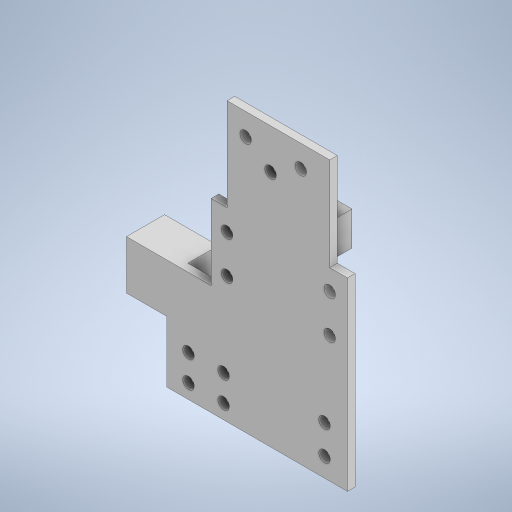
# Autodesk Inventor part: diods low holder
Saved by Autodesk Inventor 2023.1 (Build 271208000, 208)
## iProperties
Created: 2023-04-12
Part Number: diods low holder
Material: Типовые
Document SubType Name: Modeling
Designer: User
Density: 1 g/cm^3
Appearance: По умолчанию
Author: User
Autodesk Inventor part; units mm, degrees
(part 1 of 4)
ref_plane "YZ Plane" through (0, 0, 0) normal (1, 0, 0) x (0, 1, 0)
ref_plane "XZ Plane" through (0, 0, 0) normal (0, 1, 0) x (-1, 0, 0)
ref_plane "XY Plane" through (0, 0, 0) normal (0, 0, 1) x (1, 0, 0)
sketch "Эскиз1" plane through (0, 0, 0) normal (0, 0, 1) x (1, 0, 0)
  arc A0 (16.2316, 29.0119) -> (15.6959, 29.5476) centre (15.6959, 29.0119) ccw
  line L0 (15.6959, 29.5476) -> (-3.717, 29.5476)
  line L1 (-3.717, 29.5476) -> (-3.717, 30.0833)
  line L2 (-3.717, 30.0833) -> (15.6959, 30.0833)
  arc A1 (16.7673, 29.0119) -> (15.6959, 30.0833) centre (15.6959, 29.0119) ccw
  line L3 (-15.01, 19.0821) -> (-15.01, 61.0407)
  arc A2 (-14.6801, 30.0833) -> (-15.7515, 29.0119) centre (-14.6801, 29.0119) ccw
  line L4 (-14.6801, 30.0833) -> (-13.7863, 30.0833)
  line L5 (-13.7863, 30.0833) -> (-13.7863, 29.5488)
  line L6 (-13.7863, 29.5488) -> (-14.6801, 29.5488)
  arc A3 (-14.6801, 29.5488) -> (-15.217, 29.0119) centre (-14.6801, 29.0119) ccw
  arc A4 (-13.6086, 46.5113) -> (-12.5371, 45.4398) centre (-12.5371, 46.5113) ccw
  line L7 (-13.6086, 46.5113) -> (-13.6086, 48.3204)
  arc A5 (-12.5371, 49.3918) -> (-13.6086, 48.3204) centre (-12.5371, 48.3204) ccw
  line L8 (-12.5371, 49.3918) -> (13.531, 49.3918)
  arc A6 (14.6024, 48.3204) -> (13.531, 49.3918) centre (13.531, 48.3204) ccw
  line L9 (14.6024, 48.3204) -> (14.6024, 46.5113)
  arc A7 (13.531, 45.4398) -> (14.6024, 46.5113) centre (13.531, 46.5113) ccw
  line L10 (13.531, 45.4398) -> (-12.5371, 45.4398)
  arc A8 (-13.6083, 35.1179) -> (-12.5369, 34.0465) centre (-12.5369, 35.1179) ccw
  line L11 (-13.6083, 35.1179) -> (-13.6083, 43.4963)
  arc A9 (-12.5369, 44.5677) -> (-13.6083, 43.4963) centre (-12.5369, 43.4963) ccw
  line L12 (-12.5369, 44.5677) -> (13.5311, 44.5677)
  arc A10 (14.6025, 43.4963) -> (13.5311, 44.5677) centre (13.5311, 43.4963) ccw
  line L13 (14.6025, 43.4963) -> (14.6025, 35.1179)
  arc A11 (13.5311, 34.0465) -> (14.6025, 35.1179) centre (13.5311, 35.1179) ccw
  line L14 (13.5311, 34.0465) -> (-12.5369, 34.0465)
  line L15 (12.4115, -40.9097) -> (12.4115, -39.4422)
  line L16 (12.4115, -39.4422) -> (12.1037, -39.4422)
  line L17 (12.1037, -39.4422) -> (11.6041, -40.9521)
  line L18 (4.6702, -39.4422) -> (4.1371, -39.4422)
  line L19 (4.1371, -39.4422) -> (4.1371, -40.9097)
  line L20 (3.0666, -40.5083) -> (3.0666, -39.4422)
  line L21 (3.0666, -39.4422) -> (2.5335, -39.4422)
  line L22 (-3.0712, -39.3084) -> (-3.0712, -39.9752)
  line L23 (-3.0712, -39.9752) -> (-2.2727, -39.9752)
  line L24 (-2.2727, -39.9752) -> (-2.2727, -39.3084)
  line L25 (-2.2727, -40.9097) -> (-2.2727, -40.2429)
  line L26 (-2.2727, -40.2429) -> (-3.0712, -40.2429)
  line L27 (-3.0712, -40.2429) -> (-3.0712, -40.9097)
  line L28 (-8.7049, -39.3084) -> (-8.7049, -40.0957)
  line L29 (-8.7049, -40.0957) -> (-7.8573, -39.2058)
  line L30 (-7.6812, -39.4087) -> (-8.2187, -39.973)
  line L31 (-8.2187, -39.973) -> (-7.6678, -40.8227)
  line L32 (-9.7486, -40.5083) -> (-9.7486, -39.4422)
  line L33 (-9.7486, -39.4422) -> (-10.2817, -39.4422)
  line L34 (-6.4778, -35.8752) -> (-6.9921, -35.1051)
  line L35 (-6.9921, -35.1051) -> (-7.5063, -35.8752)
  line L36 (-7.7811, -35.6929) -> (-7.1907, -34.8085)
  line L37 (-7.1907, -34.8085) -> (-7.7811, -33.9242)
  line L38 (-7.5063, -33.7419) -> (-6.9921, -34.512)
  line L39 (-6.9921, -34.512) -> (-6.4778, -33.7419)
  line L40 (-6.203, -33.9242) -> (-6.7934, -34.8085)
  line L41 (-6.7934, -34.8085) -> (-6.203, -35.6929)
  line L42 (-13.0904, -31.8235) -> (-12.0092, -35.0208)
  line L43 (-12.0092, -35.0208) -> (-10.9279, -31.8235)
  line L44 (9.2465, -26.7019) -> (9.7795, -26.7019)
  line L45 (9.7795, -26.7019) -> (9.7795, -26.1689)
  line L46 (9.7795, -26.1689) -> (9.2465, -26.1689)
  line L47 (9.7795, -27.6364) -> (9.7795, -26.9696)
  line L48 (9.7795, -26.9696) -> (9.4517, -26.9696)
  line L49 (9.4517, -26.9696) -> (8.9588, -27.71)
  line L50 (7.9106, -27.235) -> (7.9106, -26.1689)
  line L51 (7.9106, -26.1689) -> (7.3775, -26.1689)
  line L52 (-0.6337, -27.6364) -> (-0.6337, -26.1689)
  line L53 (-0.6337, -26.1689) -> (-0.9414, -26.1689)
  line L54 (-0.9414, -26.1689) -> (-1.441, -27.6788)
  line L55 (-8.375, -26.1689) -> (-8.908, -26.1689)
  line L56 (-8.908, -26.1689) -> (-8.908, -27.6364)
  line L57 (-9.9785, -27.235) -> (-9.9785, -26.1689)
  line L58 (-9.9785, -26.1689) -> (-10.5116, -26.1689)
  line L59 (7.9308, 57.2595) -> (9.7846, 57.2595)
  line L60 (9.7846, 57.2595) -> (9.7846, 54.4455)
  line L61 (9.7846, 54.4455) -> (9.3105, 54.4455)
  line L62 (9.3105, 54.4455) -> (9.3105, 56.8614)
  line L63 (9.3105, 56.8614) -> (8.3441, 56.8614)
  line L64 (7.3018, 54.4455) -> (7.3018, 54.8588)
  line L65 (7.3018, 54.8588) -> (7.3261, 54.8588)
  line L66 (2.4335, 54.5883) -> (2.4335, 53.4093)
  line L67 (2.4335, 53.4093) -> (1.9594, 53.4093)
  line L68 (1.9594, 53.4093) -> (1.9594, 57.2595)
  line L69 (1.9594, 57.2595) -> (2.4335, 57.2595)
  line L70 (2.4335, 57.2595) -> (2.4335, 56.9648)
  line L71 (-1.6052, 54.4455) -> (-1.6052, 55.7127)
  line L72 (-1.6052, 55.7127) -> (-2.8755, 55.7127)
  line L73 (-2.8755, 55.7127) -> (-2.8755, 54.4455)
  line L74 (-2.8755, 54.4455) -> (-3.3496, 54.4455)
  line L75 (-3.3496, 54.4455) -> (-3.3496, 57.2595)
  line L76 (-3.3496, 57.2595) -> (-2.8755, 57.2595)
  line L77 (-2.8755, 57.2595) -> (-2.8755, 56.1199)
  line L78 (-2.8755, 56.1199) -> (-1.6052, 56.1199)
  line L79 (-1.6052, 56.1199) -> (-1.6052, 57.2595)
  line L80 (-1.6052, 57.2595) -> (-1.1312, 57.2595)
  line L81 (-1.1312, 57.2595) -> (-1.1312, 54.4455)
  line L82 (-1.1312, 54.4455) -> (-1.6052, 54.4455)
  line L83 (-1.0482, 51.8431) -> (-1.3158, 51.8431)
  line L84 (-1.3158, 51.8431) -> (-1.3158, 51.3101)
  line L85 (-1.3158, 51.3101) -> (-1.0482, 51.3101)
  line L86 (-1.3158, 52.7776) -> (-1.3158, 52.1107)
  line L87 (-1.3158, 52.1107) -> (-1.0482, 52.1107)
  line L88 (-7.1926, 51.1763) -> (-7.1926, 52.6438)
  line L89 (-7.1926, 52.6438) -> (-7.7257, 52.6438)
  line L90 (-7.7257, 52.6438) -> (-7.7257, 51.1763)
  line L91 (-6.6574, 52.6438) -> (-6.925, 52.6438)
  line L92 (-6.925, 52.6438) -> (-6.925, 51.1763)
  line L93 (-10.9306, 51.3101) -> (-10.3975, 51.3101)
  line L94 (-10.3975, 51.3101) -> (-10.3975, 52.7776)
  arc A12 (-14.7321, -26.6456) -> (-15.8036, -27.717) centre (-14.7321, -27.717) ccw
  line L95 (-14.7321, -26.6456) -> (-13.7859, -26.6456)
  line L96 (-13.7859, -26.6456) -> (-13.7859, -27.1813)
  line L97 (-13.7859, -27.1813) -> (-14.7321, -27.1813)
  arc A13 (-14.7321, -27.1813) -> (-15.2679, -27.717) centre (-14.7321, -27.717) ccw
  line L98 (-15.2679, -27.717) -> (-15.2679, -55.0248)
  arc A14 (-15.2679, -55.0248) -> (-14.7321, -55.5605) centre (-14.7321, -55.0248) ccw
  line L99 (-14.7321, -55.5605) -> (15.5357, -55.5605)
  arc A15 (15.5357, -55.5605) -> (16.0714, -55.0248) centre (15.5357, -55.0248) ccw
  line L100 (16.0714, -55.0248) -> (16.0714, -27.717)
  arc A16 (16.0714, -27.717) -> (15.5357, -27.1813) centre (15.5357, -27.717) ccw
  line L101 (15.5357, -27.1813) -> (11.1025, -27.1813)
  line L102 (11.1025, -27.1813) -> (11.1025, -26.6456)
  line L103 (11.1025, -26.6456) -> (15.5357, -26.6456)
  arc A17 (16.6071, -27.717) -> (15.5357, -26.6456) centre (15.5357, -27.717) ccw
  line L104 (16.6071, -27.717) -> (16.6071, -55.0248)
  arc A18 (15.5357, -56.0962) -> (16.6071, -55.0248) centre (15.5357, -55.0248) ccw
  line L105 (15.5357, -56.0962) -> (-14.7321, -56.0962)
  arc A19 (-15.8036, -55.0248) -> (-14.7321, -56.0962) centre (-14.7321, -55.0248) ccw
  line L106 (-15.8036, -55.0248) -> (-15.8036, -27.717)
  line L107 (-5.3214, 52.3784) -> (-5.3214, 52.1107)
  line L108 (-5.3214, 52.1107) -> (-4.523, 52.1107)
  line L109 (-4.523, 52.1107) -> (-4.523, 52.3784)
  line L110 (-4.3892, 51.8431) -> (-5.3214, 51.8431)
  line L111 (-5.3214, 51.8431) -> (-5.3214, 51.5777)
  line L112 (-2.3864, 51.1763) -> (-2.3864, 52.3628)
  line L113 (-2.3864, 52.3628) -> (-2.8101, 51.7673)
  line L114 (-3.0287, 51.7673) -> (-3.4524, 52.3628)
  line L115 (-3.4524, 52.3628) -> (-3.4524, 51.1763)
  line L116 (-3.477, 52.8557) -> (-2.9194, 52.0728)
  line L117 (-2.9194, 52.0728) -> (-2.3618, 52.8557)
  line L118 (-7.5979, 55.9407) -> (-6.4553, 54.4455)
  line L119 (-6.4553, 54.4455) -> (-7.0449, 54.4455)
  line L120 (-7.0449, 54.4455) -> (-8.0082, 55.7431)
  line L121 (-8.0082, 55.7431) -> (-8.2422, 55.7431)
  line L122 (-8.2422, 55.7431) -> (-8.2422, 54.4455)
  line L123 (-8.2422, 54.4455) -> (-8.7162, 54.4455)
  line L124 (-8.7162, 54.4455) -> (-8.7162, 57.2595)
  line L125 (-8.7162, 57.2595) -> (-8.2422, 57.2595)
  line L126 (-8.2422, 57.2595) -> (-8.2422, 56.0349)
  line L127 (-6.7774, 57.2595) -> (-6.6498, 57.2595)
  line L128 (-6.6498, 57.2595) -> (-6.6498, 56.8523)
  line L129 (-6.6498, 56.8523) -> (-6.7592, 56.8523)
  line L130 (0.6496, 56.8462) -> (0.6496, 54.4455)
  line L131 (0.6496, 54.4455) -> (0.1756, 54.4455)
  line L132 (0.1756, 54.4455) -> (0.1756, 56.8462)
  line L133 (0.1756, 56.8462) -> (-0.7817, 56.8462)
  line L134 (-0.7817, 56.8462) -> (-0.7817, 57.2595)
  line L135 (-0.7817, 57.2595) -> (1.6069, 57.2595)
  line L136 (1.6069, 57.2595) -> (1.6069, 56.8462)
  line L137 (1.6069, 56.8462) -> (0.6496, 56.8462)
  line L138 (11.2979, 55.7796) -> (10.9454, 55.7796)
  line L139 (10.9454, 55.7796) -> (10.9454, 54.8223)
  line L140 (10.9454, 54.8223) -> (11.2858, 54.8223)
  line L141 (11.456, 54.4455) -> (10.4714, 54.4455)
  line L142 (10.4714, 54.4455) -> (10.4714, 57.2595)
  line L143 (10.4714, 57.2595) -> (10.9454, 57.2595)
  line L144 (10.9454, 57.2595) -> (10.9454, 56.1625)
  line L145 (10.9454, 56.1625) -> (11.4681, 56.1625)
  line L146 (-12.646, -26.0351) -> (-12.646, -26.7019)
  line L147 (-12.646, -26.7019) -> (-11.8475, -26.7019)
  line L148 (-11.8475, -26.7019) -> (-11.8475, -26.0351)
  line L149 (-11.8475, -27.6364) -> (-11.8475, -26.9696)
  line L150 (-11.8475, -26.9696) -> (-12.646, -26.9696)
  line L151 (-12.646, -26.9696) -> (-12.646, -27.6364)
  line L152 (-6.506, -26.1689) -> (-7.039, -26.1689)
  line L153 (-7.039, -26.1689) -> (-7.039, -27.5026)
  line L154 (-7.039, -27.5026) -> (-6.506, -27.5026)
  line L155 (-6.506, -27.7703) -> (-7.039, -27.7703)
  line L156 (-7.039, -27.7703) -> (-7.039, -28.4371)
  line L157 (-4.3716, -27.235) -> (-4.3716, -26.1689)
  line L158 (-4.3716, -26.1689) -> (-4.9046, -26.1689)
  line L159 (0.7023, -26.7019) -> (1.2353, -26.7019)
  line L160 (1.2353, -26.7019) -> (1.2353, -26.1689)
  line L161 (1.2353, -26.1689) -> (0.7023, -26.1689)
  line L162 (1.2353, -27.6364) -> (1.2353, -26.9696)
  line L163 (1.2353, -26.9696) -> (0.9075, -26.9696)
  line L164 (0.9075, -26.9696) -> (0.4146, -27.71)
  line L165 (2.3059, -26.0351) -> (2.3059, -26.7019)
  line L166 (2.3059, -26.7019) -> (2.5713, -26.7019)
  line L167 (2.5713, -26.7019) -> (2.5713, -26.354)
  line L168 (2.5713, -27.3175) -> (2.5713, -26.9696)
  line L169 (2.5713, -26.9696) -> (2.3059, -26.9696)
  line L170 (2.3059, -26.9696) -> (2.3059, -27.6364)
  line L171 (5.2431, -26.0351) -> (5.2431, -27.5026)
  line L172 (5.2431, -27.5026) -> (5.7762, -27.5026)
  line L173 (5.7762, -27.5026) -> (5.7762, -26.0351)
  line L174 (6.0438, -26.0351) -> (6.0438, -27.5026)
  line L175 (6.0438, -27.5026) -> (6.1776, -27.5026)
  line L176 (6.0438, -27.9018) -> (6.0438, -27.7703)
  line L177 (6.0438, -27.7703) -> (4.7079, -27.7703)
  line L178 (4.7101, -27.5026) -> (4.9755, -27.5026)
  line L179 (4.9755, -27.5026) -> (4.9755, -26.0351)
  line L180 (-12.416, -39.3084) -> (-12.416, -39.9752)
  line L181 (-12.416, -39.9752) -> (-11.6176, -39.9752)
  line L182 (-11.6176, -39.9752) -> (-11.6176, -39.3084)
  line L183 (-11.6176, -40.9097) -> (-11.6176, -40.2429)
  line L184 (-11.6176, -40.2429) -> (-12.416, -40.2429)
  line L185 (-12.416, -40.2429) -> (-12.416, -40.9097)
  line L186 (-6.0107, -40.9097) -> (-6.0107, -39.4422)
  line L187 (-6.0107, -39.4422) -> (-6.3185, -39.4422)
  line L188 (-6.3185, -39.4422) -> (-6.818, -40.9521)
  line L189 (0.3992, -39.3084) -> (0.3992, -39.9752)
  line L190 (0.3992, -39.9752) -> (1.1976, -39.9752)
  line L191 (1.1976, -39.9752) -> (1.1976, -39.3084)
  line L192 (1.1976, -40.9097) -> (1.1976, -40.2429)
  line L193 (1.1976, -40.2429) -> (0.3992, -40.2429)
  line L194 (0.3992, -40.2429) -> (0.3992, -40.9097)
  line L195 (6.5391, -39.4422) -> (6.0061, -39.4422)
  line L196 (6.0061, -39.4422) -> (6.0061, -40.7759)
  line L197 (6.0061, -40.7759) -> (6.5391, -40.7759)
  line L198 (6.5391, -41.0435) -> (6.0061, -41.0435)
  line L199 (6.0061, -41.0435) -> (6.0061, -41.7104)
  line L200 (8.6735, -40.5083) -> (8.6735, -39.4422)
  line L201 (8.6735, -39.4422) -> (8.1405, -39.4422)
  line L202 (-5.1574, 29.8794) -> (-5.6905, 29.8794)
  line L203 (-5.6905, 29.8794) -> (-5.6905, 29.3464)
  line L204 (-5.6905, 29.3464) -> (-5.1574, 29.3464)
  line L205 (-5.6905, 30.8139) -> (-5.6905, 30.147)
  line L206 (-5.6905, 30.147) -> (-5.1574, 30.147)
  arc A20 (-14.6801, 52.299) -> (-15.7515, 51.2276) centre (-14.6801, 51.2276) ccw
  line L207 (-14.6801, 52.299) -> (-13.7863, 52.299)
  line L208 (-13.7863, 52.299) -> (-13.7863, 51.7632)
  line L209 (-13.7863, 51.7632) -> (-14.6801, 51.7632)
  arc A21 (-14.6801, 51.7632) -> (-15.2157, 51.2276) centre (-14.6801, 51.2276) ccw
  line L210 (-15.2157, 51.2276) -> (-15.2157, 33.4984)
  arc A22 (-15.2157, 33.4984) -> (-14.6801, 32.9628) centre (-14.6801, 33.4984) ccw
  line L211 (-14.6801, 32.9628) -> (15.674, 32.9628)
  arc A23 (15.674, 32.9628) -> (16.2096, 33.4984) centre (15.674, 33.4984) ccw
  line L212 (16.2096, 33.4984) -> (16.2096, 51.2276)
  arc A24 (16.2096, 51.2276) -> (15.674, 51.7632) centre (15.674, 51.2276) ccw
  line L213 (15.674, 51.7632) -> (0.7959, 51.7632)
  line L214 (0.7959, 51.7632) -> (0.7959, 52.299)
  line L215 (0.7959, 52.299) -> (15.674, 52.299)
  arc A25 (16.7454, 51.2276) -> (15.674, 52.299) centre (15.674, 51.2276) ccw
  line L216 (16.7454, 51.2276) -> (16.7454, 33.4984)
  arc A26 (15.674, 32.427) -> (16.7454, 33.4984) centre (15.674, 33.4984) ccw
  line L217 (15.674, 32.427) -> (-14.6801, 32.427)
  arc A27 (-15.7515, 33.4984) -> (-14.6801, 32.427) centre (-14.6801, 33.4984) ccw
  line L218 (-15.7515, 33.4984) -> (-15.7515, 51.2276)
  line L219 (-9.0292, 30.147) -> (-8.4962, 30.147)
  line L220 (-8.4962, 30.147) -> (-8.4962, 30.6801)
  line L221 (-8.4962, 30.6801) -> (-9.0292, 30.6801)
  line L222 (-8.4962, 29.2126) -> (-8.4962, 29.8794)
  line L223 (-8.4962, 29.8794) -> (-8.824, 29.8794)
  line L224 (-8.824, 29.8794) -> (-9.3169, 29.139)
  line L225 (0.946, -29.9199) -> (0.946, -37.6877)
  line L226 (0.946, -37.6877) -> (13.2674, -37.6877)
  line L227 (13.2674, -37.6877) -> (13.2674, -29.9199)
  line L228 (13.2674, -29.9199) -> (0.946, -29.9199)
  line L229 (0.1602, 25.5298) -> (0.1602, 17.7619)
  line L230 (0.1602, 17.7619) -> (12.4816, 17.7619)
  line L231 (12.4816, 17.7619) -> (12.4816, 25.5298)
  line L232 (12.4816, 25.5298) -> (0.1602, 25.5298)
  arc A28 (17.1429, -59.7321) -> (18.75, -58.125) centre (17.1429, -58.125) ccw
  line L233 (17.1429, -59.7321) -> (-17.1429, -59.7321)
  arc A29 (-18.75, -58.125) -> (-17.1429, -59.7321) centre (-17.1429, -58.125) ccw
  line L234 (-18.75, -58.125) -> (-18.75, 58.125)
  arc A30 (-17.1429, 59.7321) -> (-18.75, 58.125) centre (-17.1429, 58.125) ccw
  line L235 (-17.1429, 59.7321) -> (17.1429, 59.7321)
  arc A31 (18.75, 58.125) -> (17.1429, 59.7321) centre (17.1429, 58.125) ccw
  line L236 (18.75, 58.125) -> (18.75, -58.125)
  spline S0 degree 2 poles (12.5453, -41.0435) (12.4115, -41.0435) (12.4115, -40.9097) knots 0 0 0 1 1 1
  line L237 (12.5453, -41.0435) -> (12.4115, -41.0435) construction
  line L238 (12.4115, -41.0435) -> (12.4115, -40.9097) construction
  spline S1 degree 2 poles (11.6041, -40.9521) (11.5751, -41.0435) (11.4859, -41.0435) knots 0 0 0 1 1 1
  line L239 (11.6041, -40.9521) -> (11.5751, -41.0435) construction
  line L240 (11.5751, -41.0435) -> (11.4859, -41.0435) construction
  spline S2 degree 2 poles (11.4859, -41.0435) (11.3454, -41.0435) (11.3454, -40.9164) knots 0 0 0 1 1 1
  line L241 (11.4859, -41.0435) -> (11.3454, -41.0435) construction
  line L242 (11.3454, -41.0435) -> (11.3454, -40.9164) construction
  spline S3 degree 2 poles (11.3454, -40.9164) (11.3454, -40.8919) (11.3543, -40.8673) knots 0 0 0 1 1 1
  line L243 (11.3454, -40.9164) -> (11.3454, -40.8919) construction
  line L244 (11.3454, -40.8919) -> (11.3543, -40.8673) construction
  line L245 (11.3543, -40.8673) -> (11.8829, -39.266)
  spline S4 degree 2 poles (11.8829, -39.266) (11.9119, -39.1745) (12.0078, -39.1745) knots 0 0 0 1 1 1
  line L246 (11.8829, -39.266) -> (11.9119, -39.1745) construction
  line L247 (11.9119, -39.1745) -> (12.0078, -39.1745) construction
  line L248 (12.0078, -39.1745) -> (12.5453, -39.1745)
  spline S5 degree 2 poles (12.5453, -39.1745) (12.6791, -39.1745) (12.6791, -39.3084) knots 0 0 0 1 1 1
  line L249 (12.5453, -39.1745) -> (12.6791, -39.1745) construction
  line L250 (12.6791, -39.1745) -> (12.6791, -39.3084) construction
  line L251 (12.6791, -39.3084) -> (12.6791, -40.9097)
  spline S6 degree 2 poles (12.6791, -40.9097) (12.6791, -41.0435) (12.5453, -41.0435) knots 0 0 0 1 1 1
  line L252 (12.6791, -40.9097) -> (12.6791, -41.0435) construction
  line L253 (12.6791, -41.0435) -> (12.5453, -41.0435) construction
  spline S7 degree 2 poles (5.0694, -41.0435) (4.9356, -41.0435) (4.9356, -40.9097) knots 0 0 0 1 1 1
  line L254 (5.0694, -41.0435) -> (4.9356, -41.0435) construction
  line L255 (4.9356, -41.0435) -> (4.9356, -40.9097) construction
  line L256 (4.9356, -40.9097) -> (4.9356, -39.7098)
  spline S8 degree 2 poles (4.9356, -39.7098) (4.9356, -39.6005) (4.7794, -39.4422) (4.6702, -39.4422) knots 0 0 0 1 2 2 2
  line L257 (4.9356, -39.7098) -> (4.9356, -39.6005) construction
  line L258 (4.9356, -39.6005) -> (4.7794, -39.4422) construction
  line L259 (4.7794, -39.4422) -> (4.6702, -39.4422) construction
  spline S9 degree 2 poles (4.1371, -40.9097) (4.1371, -41.0435) (4.0033, -41.0435) knots 0 0 0 1 1 1
  line L260 (4.1371, -40.9097) -> (4.1371, -41.0435) construction
  line L261 (4.1371, -41.0435) -> (4.0033, -41.0435) construction
  spline S10 degree 2 poles (4.0033, -41.0435) (3.8695, -41.0435) (3.8695, -40.9097) knots 0 0 0 1 1 1
  line L262 (4.0033, -41.0435) -> (3.8695, -41.0435) construction
  line L263 (3.8695, -41.0435) -> (3.8695, -40.9097) construction
  line L264 (3.8695, -40.9097) -> (3.8695, -39.3084)
  spline S11 degree 2 poles (3.8695, -39.3084) (3.8695, -39.1745) (4.0033, -39.1745) knots 0 0 0 1 1 1
  line L265 (3.8695, -39.3084) -> (3.8695, -39.1745) construction
  line L266 (3.8695, -39.1745) -> (4.0033, -39.1745) construction
  line L267 (4.0033, -39.1745) -> (4.6702, -39.1745)
  spline S12 degree 2 poles (4.6702, -39.1745) (4.891, -39.1745) (5.2032, -39.4868) (5.2032, -39.7076) knots 0 0 0 1 2 2 2
  line L268 (4.6702, -39.1745) -> (4.891, -39.1745) construction
  line L269 (4.891, -39.1745) -> (5.2032, -39.4868) construction
  line L270 (5.2032, -39.4868) -> (5.2032, -39.7076) construction
  line L271 (5.2032, -39.7076) -> (5.2032, -40.9097)
  spline S13 degree 2 poles (5.2032, -40.9097) (5.2032, -41.0435) (5.0694, -41.0435) knots 0 0 0 1 1 1
  line L272 (5.2032, -40.9097) -> (5.2032, -41.0435) construction
  line L273 (5.2032, -41.0435) -> (5.0694, -41.0435) construction
  spline S14 degree 2 poles (2.8012, -40.7759) (2.9105, -40.7759) (3.0666, -40.6175) (3.0666, -40.5083) knots 0 0 0 1 2 2 2
  line L274 (2.8012, -40.7759) -> (2.9105, -40.7759) construction
  line L275 (2.9105, -40.7759) -> (3.0666, -40.6175) construction
  line L276 (3.0666, -40.6175) -> (3.0666, -40.5083) construction
  spline S15 degree 2 poles (2.5335, -39.4422) (2.4243, -39.4422) (2.2681, -39.6005) (2.2681, -39.7098) knots 0 0 0 1 2 2 2
  line L277 (2.5335, -39.4422) -> (2.4243, -39.4422) construction
  line L278 (2.4243, -39.4422) -> (2.2681, -39.6005) construction
  line L279 (2.2681, -39.6005) -> (2.2681, -39.7098) construction
  line L280 (2.2681, -39.7098) -> (2.2681, -40.5083)
  spline S16 degree 2 poles (2.2681, -40.5083) (2.2681, -40.6175) (2.4243, -40.7759) (2.5335, -40.7759) knots 0 0 0 1 2 2 2
  line L281 (2.2681, -40.5083) -> (2.2681, -40.6175) construction
  line L282 (2.2681, -40.6175) -> (2.4243, -40.7759) construction
  line L283 (2.4243, -40.7759) -> (2.5335, -40.7759) construction
  line L284 (2.5335, -40.7759) -> (2.8012, -40.7759)
  line L285 (2.8012, -41.0435) -> (2.5335, -41.0435)
  spline S17 degree 2 poles (2.5335, -41.0435) (2.315, -41.0435) (2.0005, -40.7313) (2.0005, -40.5105) knots 0 0 0 1 2 2 2
  line L286 (2.5335, -41.0435) -> (2.315, -41.0435) construction
  line L287 (2.315, -41.0435) -> (2.0005, -40.7313) construction
  line L288 (2.0005, -40.7313) -> (2.0005, -40.5105) construction
  line L289 (2.0005, -40.5105) -> (2.0005, -39.7076)
  spline S18 degree 2 poles (2.0005, -39.7076) (2.0005, -39.4868) (2.315, -39.1745) (2.5335, -39.1745) knots 0 0 0 1 2 2 2
  line L290 (2.0005, -39.7076) -> (2.0005, -39.4868) construction
  line L291 (2.0005, -39.4868) -> (2.315, -39.1745) construction
  line L292 (2.315, -39.1745) -> (2.5335, -39.1745) construction
  line L293 (2.5335, -39.1745) -> (3.2004, -39.1745)
  spline S19 degree 2 poles (3.2004, -39.1745) (3.3342, -39.1745) (3.3342, -39.3084) knots 0 0 0 1 1 1
  line L294 (3.2004, -39.1745) -> (3.3342, -39.1745) construction
  line L295 (3.3342, -39.1745) -> (3.3342, -39.3084) construction
  line L296 (3.3342, -39.3084) -> (3.3342, -40.506)
  spline S20 degree 2 poles (3.3342, -40.506) (3.3342, -40.7068) (3.5216, -40.787) knots 0 0 0 1 1 1
  line L297 (3.3342, -40.506) -> (3.3342, -40.7068) construction
  line L298 (3.3342, -40.7068) -> (3.5216, -40.787) construction
  spline S21 degree 2 poles (3.5216, -40.787) (3.6041, -40.8205) (3.6041, -40.9052) knots 0 0 0 1 1 1
  line L299 (3.5216, -40.787) -> (3.6041, -40.8205) construction
  line L300 (3.6041, -40.8205) -> (3.6041, -40.9052) construction
  spline S22 degree 2 poles (3.6041, -40.9052) (3.6041, -40.961) (3.5283, -41.0458) (3.4725, -41.0458) knots 0 0 0 1 2 2 2
  line L301 (3.6041, -40.9052) -> (3.6041, -40.961) construction
  line L302 (3.6041, -40.961) -> (3.5283, -41.0458) construction
  line L303 (3.5283, -41.0458) -> (3.4725, -41.0458) construction
  spline S23 degree 2 poles (3.4725, -41.0458) (3.4435, -41.0458) (3.4145, -41.0324) knots 0 0 0 1 1 1
  line L304 (3.4725, -41.0458) -> (3.4435, -41.0458) construction
  line L305 (3.4435, -41.0458) -> (3.4145, -41.0324) construction
  spline S24 degree 2 poles (3.4145, -41.0324) (3.2807, -40.9744) (3.1982, -40.8673) knots 0 0 0 1 1 1
  line L306 (3.4145, -41.0324) -> (3.2807, -40.9744) construction
  line L307 (3.2807, -40.9744) -> (3.1982, -40.8673) construction
  spline S25 degree 2 poles (3.1982, -40.8673) (3.0376, -41.0435) (2.8012, -41.0435) knots 0 0 0 1 1 1
  line L308 (3.1982, -40.8673) -> (3.0376, -41.0435) construction
  line L309 (3.0376, -41.0435) -> (2.8012, -41.0435) construction
  spline S26 degree 2 poles (-2.2727, -39.3084) (-2.2727, -39.1745) (-2.1389, -39.1745) knots 0 0 0 1 1 1
  line L310 (-2.2727, -39.3084) -> (-2.2727, -39.1745) construction
  line L311 (-2.2727, -39.1745) -> (-2.1389, -39.1745) construction
  spline S27 degree 2 poles (-2.1389, -39.1745) (-2.0051, -39.1745) (-2.0051, -39.3084) knots 0 0 0 1 1 1
  line L312 (-2.1389, -39.1745) -> (-2.0051, -39.1745) construction
  line L313 (-2.0051, -39.1745) -> (-2.0051, -39.3084) construction
  line L314 (-2.0051, -39.3084) -> (-2.0051, -40.9097)
  spline S28 degree 2 poles (-2.0051, -40.9097) (-2.0051, -41.0435) (-2.1389, -41.0435) knots 0 0 0 1 1 1
  line L315 (-2.0051, -40.9097) -> (-2.0051, -41.0435) construction
  line L316 (-2.0051, -41.0435) -> (-2.1389, -41.0435) construction
  spline S29 degree 2 poles (-2.1389, -41.0435) (-2.2727, -41.0435) (-2.2727, -40.9097) knots 0 0 0 1 1 1
  line L317 (-2.1389, -41.0435) -> (-2.2727, -41.0435) construction
  line L318 (-2.2727, -41.0435) -> (-2.2727, -40.9097) construction
  spline S30 degree 2 poles (-3.0712, -40.9097) (-3.0712, -41.0435) (-3.205, -41.0435) knots 0 0 0 1 1 1
  line L319 (-3.0712, -40.9097) -> (-3.0712, -41.0435) construction
  line L320 (-3.0712, -41.0435) -> (-3.205, -41.0435) construction
  spline S31 degree 2 poles (-3.205, -41.0435) (-3.3388, -41.0435) (-3.3388, -40.9097) knots 0 0 0 1 1 1
  line L321 (-3.205, -41.0435) -> (-3.3388, -41.0435) construction
  line L322 (-3.3388, -41.0435) -> (-3.3388, -40.9097) construction
  line L323 (-3.3388, -40.9097) -> (-3.3388, -39.3084)
  spline S32 degree 2 poles (-3.3388, -39.3084) (-3.3388, -39.1745) (-3.205, -39.1745) knots 0 0 0 1 1 1
  line L324 (-3.3388, -39.3084) -> (-3.3388, -39.1745) construction
  line L325 (-3.3388, -39.1745) -> (-3.205, -39.1745) construction
  spline S33 degree 2 poles (-3.205, -39.1745) (-3.0712, -39.1745) (-3.0712, -39.3084) knots 0 0 0 1 1 1
  line L326 (-3.205, -39.1745) -> (-3.0712, -39.1745) construction
  line L327 (-3.0712, -39.1745) -> (-3.0712, -39.3084) construction
  spline S34 degree 2 poles (-4.4606, -40.7759) (-4.3313, -40.7759) (-4.1417, -40.5885) (-4.1417, -40.4547) knots 0 0 0 1 2 2 2
  line L328 (-4.4606, -40.7759) -> (-4.3313, -40.7759) construction
  line L329 (-4.3313, -40.7759) -> (-4.1417, -40.5885) construction
  line L330 (-4.1417, -40.5885) -> (-4.1417, -40.4547) construction
  line L331 (-4.1417, -40.4547) -> (-4.1417, -39.7633)
  spline S35 degree 2 poles (-4.1417, -39.7633) (-4.1417, -39.6318) (-4.3313, -39.4422) (-4.4606, -39.4422) knots 0 0 0 1 2 2 2
  line L332 (-4.1417, -39.7633) -> (-4.1417, -39.6318) construction
  line L333 (-4.1417, -39.6318) -> (-4.3313, -39.4422) construction
  line L334 (-4.3313, -39.4422) -> (-4.4606, -39.4422) construction
  line L335 (-4.4606, -39.4422) -> (-4.6212, -39.4422)
  spline S36 degree 2 poles (-4.6212, -39.4422) (-4.7528, -39.4422) (-4.9401, -39.6318) (-4.9401, -39.7633) knots 0 0 0 1 2 2 2
  line L336 (-4.6212, -39.4422) -> (-4.7528, -39.4422) construction
  line L337 (-4.7528, -39.4422) -> (-4.9401, -39.6318) construction
  line L338 (-4.9401, -39.6318) -> (-4.9401, -39.7633) construction
  line L339 (-4.9401, -39.7633) -> (-4.9401, -40.4547)
  spline S37 degree 2 poles (-4.9401, -40.4547) (-4.9401, -40.5885) (-4.7528, -40.7759) (-4.6212, -40.7759) knots 0 0 0 1 2 2 2
  line L340 (-4.9401, -40.4547) -> (-4.9401, -40.5885) construction
  line L341 (-4.9401, -40.5885) -> (-4.7528, -40.7759) construction
  line L342 (-4.7528, -40.7759) -> (-4.6212, -40.7759) construction
  line L343 (-4.6212, -40.7759) -> (-4.4606, -40.7759)
  line L344 (-4.4606, -41.0435) -> (-4.6212, -41.0435)
  spline S38 degree 2 poles (-4.6212, -41.0435) (-4.8621, -41.0435) (-5.2078, -40.7001) (-5.2078, -40.457) knots 0 0 0 1 2 2 2
  line L345 (-4.6212, -41.0435) -> (-4.8621, -41.0435) construction
  line L346 (-4.8621, -41.0435) -> (-5.2078, -40.7001) construction
  line L347 (-5.2078, -40.7001) -> (-5.2078, -40.457) construction
  line L348 (-5.2078, -40.457) -> (-5.2078, -39.7611)
  spline S39 degree 2 poles (-5.2078, -39.7611) (-5.2078, -39.518) (-4.8621, -39.1745) (-4.6212, -39.1745) knots 0 0 0 1 2 2 2
  line L349 (-5.2078, -39.7611) -> (-5.2078, -39.518) construction
  line L350 (-5.2078, -39.518) -> (-4.8621, -39.1745) construction
  line L351 (-4.8621, -39.1745) -> (-4.6212, -39.1745) construction
  line L352 (-4.6212, -39.1745) -> (-4.4606, -39.1745)
  spline S40 degree 2 poles (-4.4606, -39.1745) (-4.2175, -39.1745) (-3.8741, -39.518) (-3.8741, -39.7611) knots 0 0 0 1 2 2 2
  line L353 (-4.4606, -39.1745) -> (-4.2175, -39.1745) construction
  line L354 (-4.2175, -39.1745) -> (-3.8741, -39.518) construction
  line L355 (-3.8741, -39.518) -> (-3.8741, -39.7611) construction
  line L356 (-3.8741, -39.7611) -> (-3.8741, -40.457)
  spline S41 degree 2 poles (-3.8741, -40.457) (-3.8741, -40.7023) (-4.2175, -41.0435) (-4.4606, -41.0435) knots 0 0 0 1 2 2 2
  line L357 (-3.8741, -40.457) -> (-3.8741, -40.7023) construction
  line L358 (-3.8741, -40.7023) -> (-4.2175, -41.0435) construction
  line L359 (-4.2175, -41.0435) -> (-4.4606, -41.0435) construction
  line L360 (-8.7049, -40.4837) -> (-8.7049, -40.9097)
  spline S42 degree 2 poles (-8.7049, -40.9097) (-8.7049, -41.0435) (-8.8387, -41.0435) knots 0 0 0 1 1 1
  line L361 (-8.7049, -40.9097) -> (-8.7049, -41.0435) construction
  line L362 (-8.7049, -41.0435) -> (-8.8387, -41.0435) construction
  spline S43 degree 2 poles (-8.8387, -41.0435) (-8.9725, -41.0435) (-8.9725, -40.9097) knots 0 0 0 1 1 1
  line L363 (-8.8387, -41.0435) -> (-8.9725, -41.0435) construction
  line L364 (-8.9725, -41.0435) -> (-8.9725, -40.9097) construction
  line L365 (-8.9725, -40.9097) -> (-8.9725, -39.3084)
  spline S44 degree 2 poles (-8.9725, -39.3084) (-8.9725, -39.1745) (-8.8387, -39.1745) knots 0 0 0 1 1 1
  line L366 (-8.9725, -39.3084) -> (-8.9725, -39.1745) construction
  line L367 (-8.9725, -39.1745) -> (-8.8387, -39.1745) construction
  spline S45 degree 2 poles (-8.8387, -39.1745) (-8.7049, -39.1745) (-8.7049, -39.3084) knots 0 0 0 1 1 1
  line L368 (-8.8387, -39.1745) -> (-8.7049, -39.1745) construction
  line L369 (-8.7049, -39.1745) -> (-8.7049, -39.3084) construction
  spline S46 degree 2 poles (-7.8573, -39.2058) (-7.8217, -39.1656) (-7.7726, -39.1656) knots 0 0 0 1 1 1
  line L370 (-7.8573, -39.2058) -> (-7.8217, -39.1656) construction
  line L371 (-7.8217, -39.1656) -> (-7.7726, -39.1656) construction
  spline S47 degree 2 poles (-7.7726, -39.1656) (-7.7191, -39.1656) (-7.6388, -39.2526) (-7.6388, -39.3106) knots 0 0 0 1 2 2 2
  line L372 (-7.7726, -39.1656) -> (-7.7191, -39.1656) construction
  line L373 (-7.7191, -39.1656) -> (-7.6388, -39.2526) construction
  line L374 (-7.6388, -39.2526) -> (-7.6388, -39.3106) construction
  spline S48 degree 2 poles (-7.6388, -39.3106) (-7.6388, -39.3664) (-7.6812, -39.4087) knots 0 0 0 1 1 1
  line L375 (-7.6388, -39.3106) -> (-7.6388, -39.3664) construction
  line L376 (-7.6388, -39.3664) -> (-7.6812, -39.4087) construction
  spline S49 degree 2 poles (-7.6678, -40.8227) (-7.6388, -40.8673) (-7.6388, -40.9119) knots 0 0 0 1 1 1
  line L377 (-7.6678, -40.8227) -> (-7.6388, -40.8673) construction
  line L378 (-7.6388, -40.8673) -> (-7.6388, -40.9119) construction
  spline S50 degree 2 poles (-7.6388, -40.9119) (-7.6388, -40.9677) (-7.7258, -41.048) (-7.7748, -41.048) knots 0 0 0 1 2 2 2
  line L379 (-7.6388, -40.9119) -> (-7.6388, -40.9677) construction
  line L380 (-7.6388, -40.9677) -> (-7.7258, -41.048) construction
  line L381 (-7.7258, -41.048) -> (-7.7748, -41.048) construction
  spline S51 degree 2 poles (-7.7748, -41.048) (-7.8373, -41.048) (-7.8707, -40.9945) knots 0 0 0 1 1 1
  line L382 (-7.7748, -41.048) -> (-7.8373, -41.048) construction
  line L383 (-7.8373, -41.048) -> (-7.8707, -40.9945) construction
  line L384 (-7.8707, -40.9945) -> (-8.406, -40.1693)
  spline S52 degree 2 poles (-8.406, -40.1693) (-8.4863, -40.254) (-8.7049, -40.4837) knots 0 0 0 1 1 1
  line L385 (-8.406, -40.1693) -> (-8.4863, -40.254) construction
  line L386 (-8.4863, -40.254) -> (-8.7049, -40.4837) construction
  spline S53 degree 2 poles (-10.014, -40.7759) (-9.9047, -40.7759) (-9.7486, -40.6175) (-9.7486, -40.5083) knots 0 0 0 1 2 2 2
  line L387 (-10.014, -40.7759) -> (-9.9047, -40.7759) construction
  line L388 (-9.9047, -40.7759) -> (-9.7486, -40.6175) construction
  line L389 (-9.7486, -40.6175) -> (-9.7486, -40.5083) construction
  spline S54 degree 2 poles (-10.2817, -39.4422) (-10.391, -39.4422) (-10.5471, -39.6005) (-10.5471, -39.7098) knots 0 0 0 1 2 2 2
  line L390 (-10.2817, -39.4422) -> (-10.391, -39.4422) construction
  line L391 (-10.391, -39.4422) -> (-10.5471, -39.6005) construction
  line L392 (-10.5471, -39.6005) -> (-10.5471, -39.7098) construction
  line L393 (-10.5471, -39.7098) -> (-10.5471, -40.5083)
  spline S55 degree 2 poles (-10.5471, -40.5083) (-10.5471, -40.6175) (-10.391, -40.7759) (-10.2817, -40.7759) knots 0 0 0 1 2 2 2
  line L394 (-10.5471, -40.5083) -> (-10.5471, -40.6175) construction
  line L395 (-10.5471, -40.6175) -> (-10.391, -40.7759) construction
  line L396 (-10.391, -40.7759) -> (-10.2817, -40.7759) construction
  line L397 (-10.2817, -40.7759) -> (-10.014, -40.7759)
  line L398 (-10.014, -41.0435) -> (-10.2817, -41.0435)
  spline S56 degree 2 poles (-10.2817, -41.0435) (-10.5002, -41.0435) (-10.8147, -40.7313) (-10.8147, -40.5105) knots 0 0 0 1 2 2 2
  line L399 (-10.2817, -41.0435) -> (-10.5002, -41.0435) construction
  line L400 (-10.5002, -41.0435) -> (-10.8147, -40.7313) construction
  line L401 (-10.8147, -40.7313) -> (-10.8147, -40.5105) construction
  line L402 (-10.8147, -40.5105) -> (-10.8147, -39.7076)
  spline S57 degree 2 poles (-10.8147, -39.7076) (-10.8147, -39.4868) (-10.5002, -39.1745) (-10.2817, -39.1745) knots 0 0 0 1 2 2 2
  line L403 (-10.8147, -39.7076) -> (-10.8147, -39.4868) construction
  line L404 (-10.8147, -39.4868) -> (-10.5002, -39.1745) construction
  line L405 (-10.5002, -39.1745) -> (-10.2817, -39.1745) construction
  line L406 (-10.2817, -39.1745) -> (-9.6148, -39.1745)
  spline S58 degree 2 poles (-9.6148, -39.1745) (-9.481, -39.1745) (-9.481, -39.3084) knots 0 0 0 1 1 1
  line L407 (-9.6148, -39.1745) -> (-9.481, -39.1745) construction
  line L408 (-9.481, -39.1745) -> (-9.481, -39.3084) construction
  line L409 (-9.481, -39.3084) -> (-9.481, -40.506)
  spline S59 degree 2 poles (-9.481, -40.506) (-9.481, -40.7068) (-9.2937, -40.787) knots 0 0 0 1 1 1
  line L410 (-9.481, -40.506) -> (-9.481, -40.7068) construction
  line L411 (-9.481, -40.7068) -> (-9.2937, -40.787) construction
  spline S60 degree 2 poles (-9.2937, -40.787) (-9.2111, -40.8205) (-9.2111, -40.9052) knots 0 0 0 1 1 1
  line L412 (-9.2937, -40.787) -> (-9.2111, -40.8205) construction
  line L413 (-9.2111, -40.8205) -> (-9.2111, -40.9052) construction
  spline S61 degree 2 poles (-9.2111, -40.9052) (-9.2111, -40.961) (-9.287, -41.0458) (-9.3427, -41.0458) knots 0 0 0 1 2 2 2
  line L414 (-9.2111, -40.9052) -> (-9.2111, -40.961) construction
  line L415 (-9.2111, -40.961) -> (-9.287, -41.0458) construction
  line L416 (-9.287, -41.0458) -> (-9.3427, -41.0458) construction
  spline S62 degree 2 poles (-9.3427, -41.0458) (-9.3717, -41.0458) (-9.4007, -41.0324) knots 0 0 0 1 1 1
  line L417 (-9.3427, -41.0458) -> (-9.3717, -41.0458) construction
  line L418 (-9.3717, -41.0458) -> (-9.4007, -41.0324) construction
  spline S63 degree 2 poles (-9.4007, -41.0324) (-9.5345, -40.9744) (-9.617, -40.8673) knots 0 0 0 1 1 1
  line L419 (-9.4007, -41.0324) -> (-9.5345, -40.9744) construction
  line L420 (-9.5345, -40.9744) -> (-9.617, -40.8673) construction
  spline S64 degree 2 poles (-9.617, -40.8673) (-9.7776, -41.0435) (-10.014, -41.0435) knots 0 0 0 1 1 1
  line L421 (-9.617, -40.8673) -> (-9.7776, -41.0435) construction
  line L422 (-9.7776, -41.0435) -> (-10.014, -41.0435) construction
  spline S65 degree 2 poles (-3.0954, -33.5444) (-3.3631, -33.5444) (-3.3631, -33.2767) knots 0 0 0 1 1 1
  line L423 (-3.0954, -33.5444) -> (-3.3631, -33.5444) construction
  line L424 (-3.3631, -33.5444) -> (-3.3631, -33.2767) construction
  spline S66 degree 2 poles (-3.3631, -33.2767) (-3.3631, -33.0091) (-3.0954, -33.0091) knots 0 0 0 1 1 1
  line L425 (-3.3631, -33.2767) -> (-3.3631, -33.0091) construction
  line L426 (-3.3631, -33.0091) -> (-3.0954, -33.0091) construction
  line L427 (-3.0954, -33.0091) -> (-0.9588, -33.0091)
  spline S67 degree 2 poles (-0.9588, -33.0091) (-0.6957, -33.0091) (-0.6957, -33.2767) knots 0 0 0 1 1 1
  line L428 (-0.9588, -33.0091) -> (-0.6957, -33.0091) construction
  line L429 (-0.6957, -33.0091) -> (-0.6957, -33.2767) construction
  spline S68 degree 2 poles (-0.6957, -33.2767) (-0.6957, -33.5444) (-0.9588, -33.5444) knots 0 0 0 1 1 1
  line L430 (-0.6957, -33.2767) -> (-0.6957, -33.5444) construction
  line L431 (-0.6957, -33.5444) -> (-0.9588, -33.5444) construction
  line L432 (-0.9588, -33.5444) -> (-3.0954, -33.5444)
  spline S69 degree 2 poles (-6.3472, -35.9513) (-6.4288, -35.9513) (-6.4778, -35.8752) knots 0 0 0 1 1 1
  line L433 (-6.3472, -35.9513) -> (-6.4288, -35.9513) construction
  line L434 (-6.4288, -35.9513) -> (-6.4778, -35.8752) construction
  spline S70 degree 2 poles (-7.5063, -35.8752) (-7.5553, -35.9513) (-7.6369, -35.9513) knots 0 0 0 1 1 1
  line L435 (-7.5063, -35.8752) -> (-7.5553, -35.9513) construction
  line L436 (-7.5553, -35.9513) -> (-7.6369, -35.9513) construction
  spline S71 degree 2 poles (-7.6369, -35.9513) (-7.7022, -35.9513) (-7.8083, -35.8534) (-7.8083, -35.7854) knots 0 0 0 1 2 2 2
  line L437 (-7.6369, -35.9513) -> (-7.7022, -35.9513) construction
  line L438 (-7.7022, -35.9513) -> (-7.8083, -35.8534) construction
  line L439 (-7.8083, -35.8534) -> (-7.8083, -35.7854) construction
  spline S72 degree 2 poles (-7.8083, -35.7854) (-7.8083, -35.7391) (-7.7811, -35.6929) knots 0 0 0 1 1 1
  line L440 (-7.8083, -35.7854) -> (-7.8083, -35.7391) construction
  line L441 (-7.8083, -35.7391) -> (-7.7811, -35.6929) construction
  spline S73 degree 2 poles (-7.7811, -33.9242) (-7.8083, -33.878) (-7.8083, -33.8317) knots 0 0 0 1 1 1
  line L442 (-7.7811, -33.9242) -> (-7.8083, -33.878) construction
  line L443 (-7.8083, -33.878) -> (-7.8083, -33.8317) construction
  spline S74 degree 2 poles (-7.8083, -33.8317) (-7.8083, -33.7637) (-7.7022, -33.6658) (-7.6369, -33.6658) knots 0 0 0 1 2 2 2
  line L444 (-7.8083, -33.8317) -> (-7.8083, -33.7637) construction
  line L445 (-7.8083, -33.7637) -> (-7.7022, -33.6658) construction
  line L446 (-7.7022, -33.6658) -> (-7.6369, -33.6658) construction
  spline S75 degree 2 poles (-7.6369, -33.6658) (-7.5553, -33.6658) (-7.5063, -33.7419) knots 0 0 0 1 1 1
  line L447 (-7.6369, -33.6658) -> (-7.5553, -33.6658) construction
  line L448 (-7.5553, -33.6658) -> (-7.5063, -33.7419) construction
  spline S76 degree 2 poles (-6.4778, -33.7419) (-6.4288, -33.6658) (-6.3472, -33.6658) knots 0 0 0 1 1 1
  line L449 (-6.4778, -33.7419) -> (-6.4288, -33.6658) construction
  line L450 (-6.4288, -33.6658) -> (-6.3472, -33.6658) construction
  spline S77 degree 2 poles (-6.3472, -33.6658) (-6.2819, -33.6658) (-6.1731, -33.7637) (-6.1731, -33.8317) knots 0 0 0 1 2 2 2
  line L451 (-6.3472, -33.6658) -> (-6.2819, -33.6658) construction
  line L452 (-6.2819, -33.6658) -> (-6.1731, -33.7637) construction
  line L453 (-6.1731, -33.7637) -> (-6.1731, -33.8317) construction
  spline S78 degree 2 poles (-6.1731, -33.8317) (-6.1731, -33.878) (-6.203, -33.9242) knots 0 0 0 1 1 1
  line L454 (-6.1731, -33.8317) -> (-6.1731, -33.878) construction
  line L455 (-6.1731, -33.878) -> (-6.203, -33.9242) construction
  spline S79 degree 2 poles (-6.203, -35.6929) (-6.1731, -35.7391) (-6.1731, -35.7854) knots 0 0 0 1 1 1
  line L456 (-6.203, -35.6929) -> (-6.1731, -35.7391) construction
  line L457 (-6.1731, -35.7391) -> (-6.1731, -35.7854) construction
  spline S80 degree 2 poles (-6.1731, -35.7854) (-6.1731, -35.8534) (-6.2819, -35.9513) (-6.3472, -35.9513) knots 0 0 0 1 2 2 2
  line L458 (-6.1731, -35.7854) -> (-6.1731, -35.8534) construction
  line L459 (-6.1731, -35.8534) -> (-6.2819, -35.9513) construction
  line L460 (-6.2819, -35.9513) -> (-6.3472, -35.9513) construction
  spline S81 degree 2 poles (-11.8093, -35.7631) (-11.87, -35.9451) (-12.0092, -35.9451) knots 0 0 0 1 1 1
  line L461 (-11.8093, -35.7631) -> (-11.87, -35.9451) construction
  line L462 (-11.87, -35.9451) -> (-12.0092, -35.9451) construction
  spline S82 degree 2 poles (-12.0092, -35.9451) (-12.1519, -35.9451) (-12.209, -35.7631) knots 0 0 0 1 1 1
  line L463 (-12.0092, -35.9451) -> (-12.1519, -35.9451) construction
  line L464 (-12.1519, -35.9451) -> (-12.209, -35.7631) construction
  line L465 (-12.209, -35.7631) -> (-13.4937, -31.9591)
  spline S83 degree 2 poles (-13.4937, -31.9591) (-13.5044, -31.9198) (-13.5044, -31.8806) knots 0 0 0 1 1 1
  line L466 (-13.4937, -31.9591) -> (-13.5044, -31.9198) construction
  line L467 (-13.5044, -31.9198) -> (-13.5044, -31.8806) construction
  spline S84 degree 2 poles (-13.5044, -31.8806) (-13.5044, -31.6772) (-13.2831, -31.6772) knots 0 0 0 1 1 1
  line L468 (-13.5044, -31.8806) -> (-13.5044, -31.6772) construction
  line L469 (-13.5044, -31.6772) -> (-13.2831, -31.6772) construction
  spline S85 degree 2 poles (-13.2831, -31.6772) (-13.1404, -31.6772) (-13.0904, -31.8235) knots 0 0 0 1 1 1
  line L470 (-13.2831, -31.6772) -> (-13.1404, -31.6772) construction
  line L471 (-13.1404, -31.6772) -> (-13.0904, -31.8235) construction
  spline S86 degree 2 poles (-10.9279, -31.8235) (-10.878, -31.6772) (-10.7352, -31.6772) knots 0 0 0 1 1 1
  line L472 (-10.9279, -31.8235) -> (-10.878, -31.6772) construction
  line L473 (-10.878, -31.6772) -> (-10.7352, -31.6772) construction
  spline S87 degree 2 poles (-10.7352, -31.6772) (-10.514, -31.6772) (-10.514, -31.8806) knots 0 0 0 1 1 1
  line L474 (-10.7352, -31.6772) -> (-10.514, -31.6772) construction
  line L475 (-10.514, -31.6772) -> (-10.514, -31.8806) construction
  spline S88 degree 2 poles (-10.514, -31.8806) (-10.514, -31.9198) (-10.5283, -31.9591) knots 0 0 0 1 1 1
  line L476 (-10.514, -31.8806) -> (-10.514, -31.9198) construction
  line L477 (-10.514, -31.9198) -> (-10.5283, -31.9591) construction
  line L478 (-10.5283, -31.9591) -> (-11.8093, -35.7631)
  spline S89 degree 2 poles (9.2465, -26.1689) (9.1216, -26.1689) (8.9811, -26.325) (8.9811, -26.4343) knots 0 0 0 1 2 2 2
  line L479 (9.2465, -26.1689) -> (9.1216, -26.1689) construction
  line L480 (9.1216, -26.1689) -> (8.9811, -26.325) construction
  line L481 (8.9811, -26.325) -> (8.9811, -26.4343) construction
  spline S90 degree 2 poles (8.9811, -26.4343) (8.9811, -26.5436) (9.048, -26.6194) knots 0 0 0 1 1 1
  line L482 (8.9811, -26.4343) -> (8.9811, -26.5436) construction
  line L483 (8.9811, -26.5436) -> (9.048, -26.6194) construction
  spline S91 degree 2 poles (9.048, -26.6194) (9.1216, -26.7019) (9.2465, -26.7019) knots 0 0 0 1 1 1
  line L484 (9.048, -26.6194) -> (9.1216, -26.7019) construction
  line L485 (9.1216, -26.7019) -> (9.2465, -26.7019) construction
  spline S92 degree 2 poles (8.9588, -27.71) (8.9187, -27.7725) (8.8517, -27.7725) knots 0 0 0 1 1 1
  line L486 (8.9588, -27.71) -> (8.9187, -27.7725) construction
  line L487 (8.9187, -27.7725) -> (8.8517, -27.7725) construction
  spline S93 degree 2 poles (8.8517, -27.7725) (8.796, -27.7725) (8.7112, -27.6922) (8.7112, -27.6387) knots 0 0 0 1 2 2 2
  line L488 (8.8517, -27.7725) -> (8.796, -27.7725) construction
  line L489 (8.796, -27.7725) -> (8.7112, -27.6922) construction
  line L490 (8.7112, -27.6922) -> (8.7112, -27.6387) construction
  spline S94 degree 2 poles (8.7112, -27.6387) (8.7112, -27.5985) (8.7358, -27.5628) knots 0 0 0 1 1 1
  line L491 (8.7112, -27.6387) -> (8.7112, -27.5985) construction
  line L492 (8.7112, -27.5985) -> (8.7358, -27.5628) construction
  line L493 (8.7358, -27.5628) -> (9.1372, -26.9607)
  spline S95 degree 2 poles (9.1372, -26.9607) (8.9365, -26.9272) (8.8183, -26.7689) knots 0 0 0 1 1 1
  line L494 (9.1372, -26.9607) -> (8.9365, -26.9272) construction
  line L495 (8.9365, -26.9272) -> (8.8183, -26.7689) construction
  spline S96 degree 2 poles (8.8183, -26.7689) (8.7135, -26.6261) (8.7135, -26.4343) knots 0 0 0 1 1 1
  line L496 (8.8183, -26.7689) -> (8.7135, -26.6261) construction
  line L497 (8.7135, -26.6261) -> (8.7135, -26.4343) construction
  spline S97 degree 2 poles (8.7135, -26.4343) (8.7135, -26.218) (8.8473, -26.0685) knots 0 0 0 1 1 1
  line L498 (8.7135, -26.4343) -> (8.7135, -26.218) construction
  line L499 (8.7135, -26.218) -> (8.8473, -26.0685) construction
  spline S98 degree 2 poles (8.8473, -26.0685) (8.9945, -25.9013) (9.2465, -25.9013) knots 0 0 0 1 1 1
  line L500 (8.8473, -26.0685) -> (8.9945, -25.9013) construction
  line L501 (8.9945, -25.9013) -> (9.2465, -25.9013) construction
  line L502 (9.2465, -25.9013) -> (9.9134, -25.9013)
  spline S99 degree 2 poles (9.9134, -25.9013) (10.0472, -25.9013) (10.0472, -26.0351) knots 0 0 0 1 1 1
  line L503 (9.9134, -25.9013) -> (10.0472, -25.9013) construction
  line L504 (10.0472, -25.9013) -> (10.0472, -26.0351) construction
  line L505 (10.0472, -26.0351) -> (10.0472, -27.6364)
  spline S100 degree 2 poles (10.0472, -27.6364) (10.0472, -27.7703) (9.9134, -27.7703) knots 0 0 0 1 1 1
  line L506 (10.0472, -27.6364) -> (10.0472, -27.7703) construction
  line L507 (10.0472, -27.7703) -> (9.9134, -27.7703) construction
  spline S101 degree 2 poles (9.9134, -27.7703) (9.7795, -27.7703) (9.7795, -27.6364) knots 0 0 0 1 1 1
  line L508 (9.9134, -27.7703) -> (9.7795, -27.7703) construction
  line L509 (9.7795, -27.7703) -> (9.7795, -27.6364) construction
  spline S102 degree 2 poles (7.6452, -27.5026) (7.7544, -27.5026) (7.9106, -27.3443) (7.9106, -27.235) knots 0 0 0 1 2 2 2
  line L510 (7.6452, -27.5026) -> (7.7544, -27.5026) construction
  line L511 (7.7544, -27.5026) -> (7.9106, -27.3443) construction
  line L512 (7.9106, -27.3443) -> (7.9106, -27.235) construction
  spline S103 degree 2 poles (7.3775, -26.1689) (7.2682, -26.1689) (7.1121, -26.3273) (7.1121, -26.4365) knots 0 0 0 1 2 2 2
  line L513 (7.3775, -26.1689) -> (7.2682, -26.1689) construction
  line L514 (7.2682, -26.1689) -> (7.1121, -26.3273) construction
  line L515 (7.1121, -26.3273) -> (7.1121, -26.4365) construction
  line L516 (7.1121, -26.4365) -> (7.1121, -27.235)
  spline S104 degree 2 poles (7.1121, -27.235) (7.1121, -27.3443) (7.2682, -27.5026) (7.3775, -27.5026) knots 0 0 0 1 2 2 2
  line L517 (7.1121, -27.235) -> (7.1121, -27.3443) construction
  line L518 (7.1121, -27.3443) -> (7.2682, -27.5026) construction
  line L519 (7.2682, -27.5026) -> (7.3775, -27.5026) construction
  line L520 (7.3775, -27.5026) -> (7.6452, -27.5026)
  line L521 (7.6452, -27.7703) -> (7.3775, -27.7703)
  spline S105 degree 2 poles (7.3775, -27.7703) (7.159, -27.7703) (6.8445, -27.458) (6.8445, -27.2372) knots 0 0 0 1 2 2 2
  line L522 (7.3775, -27.7703) -> (7.159, -27.7703) construction
  line L523 (7.159, -27.7703) -> (6.8445, -27.458) construction
  line L524 (6.8445, -27.458) -> (6.8445, -27.2372) construction
  line L525 (6.8445, -27.2372) -> (6.8445, -26.4343)
  spline S106 degree 2 poles (6.8445, -26.4343) (6.8445, -26.2135) (7.159, -25.9013) (7.3775, -25.9013) knots 0 0 0 1 2 2 2
  line L526 (6.8445, -26.4343) -> (6.8445, -26.2135) construction
  line L527 (6.8445, -26.2135) -> (7.159, -25.9013) construction
  line L528 (7.159, -25.9013) -> (7.3775, -25.9013) construction
  line L529 (7.3775, -25.9013) -> (8.0444, -25.9013)
  spline S107 degree 2 poles (8.0444, -25.9013) (8.1782, -25.9013) (8.1782, -26.0351) knots 0 0 0 1 1 1
  line L530 (8.0444, -25.9013) -> (8.1782, -25.9013) construction
  line L531 (8.1782, -25.9013) -> (8.1782, -26.0351) construction
  line L532 (8.1782, -26.0351) -> (8.1782, -27.2328)
  spline S108 degree 2 poles (8.1782, -27.2328) (8.1782, -27.4335) (8.3655, -27.5138) knots 0 0 0 1 1 1
  line L533 (8.1782, -27.2328) -> (8.1782, -27.4335) construction
  line L534 (8.1782, -27.4335) -> (8.3655, -27.5138) construction
  spline S109 degree 2 poles (8.3655, -27.5138) (8.4481, -27.5472) (8.4481, -27.632) knots 0 0 0 1 1 1
  line L535 (8.3655, -27.5138) -> (8.4481, -27.5472) construction
  line L536 (8.4481, -27.5472) -> (8.4481, -27.632) construction
  spline S110 degree 2 poles (8.4481, -27.632) (8.4481, -27.6877) (8.3722, -27.7725) (8.3165, -27.7725) knots 0 0 0 1 2 2 2
  line L537 (8.4481, -27.632) -> (8.4481, -27.6877) construction
  line L538 (8.4481, -27.6877) -> (8.3722, -27.7725) construction
  line L539 (8.3722, -27.7725) -> (8.3165, -27.7725) construction
  spline S111 degree 2 poles (8.3165, -27.7725) (8.2875, -27.7725) (8.2585, -27.7591) knots 0 0 0 1 1 1
  line L540 (8.3165, -27.7725) -> (8.2875, -27.7725) construction
  line L541 (8.2875, -27.7725) -> (8.2585, -27.7591) construction
  spline S112 degree 2 poles (8.2585, -27.7591) (8.1247, -27.7011) (8.0422, -27.5941) knots 0 0 0 1 1 1
  line L542 (8.2585, -27.7591) -> (8.1247, -27.7011) construction
  line L543 (8.1247, -27.7011) -> (8.0422, -27.5941) construction
  spline S113 degree 2 poles (8.0422, -27.5941) (7.8816, -27.7703) (7.6452, -27.7703) knots 0 0 0 1 1 1
  line L544 (8.0422, -27.5941) -> (7.8816, -27.7703) construction
  line L545 (7.8816, -27.7703) -> (7.6452, -27.7703) construction
  spline S114 degree 2 poles (-0.4998, -27.7703) (-0.6337, -27.7703) (-0.6337, -27.6364) knots 0 0 0 1 1 1
  line L546 (-0.4998, -27.7703) -> (-0.6337, -27.7703) construction
  line L547 (-0.6337, -27.7703) -> (-0.6337, -27.6364) construction
  spline S115 degree 2 poles (-1.441, -27.6788) (-1.47, -27.7703) (-1.5592, -27.7703) knots 0 0 0 1 1 1
  line L548 (-1.441, -27.6788) -> (-1.47, -27.7703) construction
  line L549 (-1.47, -27.7703) -> (-1.5592, -27.7703) construction
  spline S116 degree 2 poles (-1.5592, -27.7703) (-1.6997, -27.7703) (-1.6997, -27.6431) knots 0 0 0 1 1 1
  line L550 (-1.5592, -27.7703) -> (-1.6997, -27.7703) construction
  line L551 (-1.6997, -27.7703) -> (-1.6997, -27.6431) construction
  spline S117 degree 2 poles (-1.6997, -27.6431) (-1.6997, -27.6186) (-1.6908, -27.5941) knots 0 0 0 1 1 1
  line L552 (-1.6997, -27.6431) -> (-1.6997, -27.6186) construction
  line L553 (-1.6997, -27.6186) -> (-1.6908, -27.5941) construction
  line L554 (-1.6908, -27.5941) -> (-1.1622, -25.9927)
  spline S118 degree 2 poles (-1.1622, -25.9927) (-1.1332, -25.9013) (-1.0373, -25.9013) knots 0 0 0 1 1 1
  line L555 (-1.1622, -25.9927) -> (-1.1332, -25.9013) construction
  line L556 (-1.1332, -25.9013) -> (-1.0373, -25.9013) construction
  line L557 (-1.0373, -25.9013) -> (-0.4998, -25.9013)